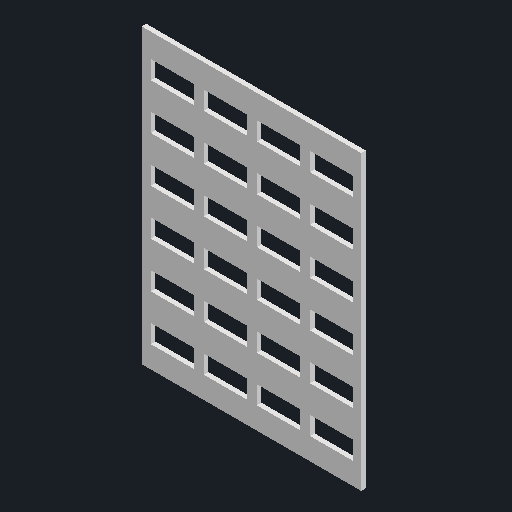
# Autodesk Inventor part: Base
Saved by Autodesk Inventor 2026.1 (Build 301233000, 233)
## iProperties
Created: 2026-06-15
Part Number: Base
Material: Generic
Document SubType Name: Modeling
Designer: aleja
Density: 1 g/cm^3
Appearance: Default
Author: aleja
Autodesk Inventor part; units mm, degrees
ref_plane "YZ Plane" through (0, 0, 0) normal (1, 0, 0) x (0, 1, 0)
ref_plane "XZ Plane" through (0, 0, 0) normal (0, 1, 0) x (-1, 0, 0)
ref_plane "XY Plane" through (0, 0, 0) normal (0, 0, 1) x (1, 0, 0)
sketch "Sketch1" plane through (0, 0, 0) normal (0, 1, 0) x (-1, 0, 0)
  line L0 (-60, 80) -> (60, 80)
  line L1 (60, 80) -> (60, -80)
  line L2 (60, -80) -> (-60, -80)
  line L3 (-60, -80) -> (-60, 80)
  line L4 (-60, 80) -> (60, -80) construction
  line L5 (60, 80) -> (-60, -80) construction
  point P0 (0, 0)
  dimension "d0" = 160
  dimension "d1" = 120
  constraints: 12 end point, 2 midpoint, 2 parallel, 1 horizontal, 1 perpendicular
  measures "d0" distance of L0.end L1.end
  measures "d1" distance of L1.end L2.end
extrude "Extrusion1" add sketch "Sketch1" along normal blind 5
sketch "Sketch2" plane through (60, 0, 80) normal (1, 0, 0) x (0, 0, -1)
  line L0 (0, 0) -> (0, 5) projected
  line L1 (0, 0) -> (0, 5) projected
  line L2 (0, 0) -> (160, 0) projected
  line L3 (160, 0) -> (160, 5) projected
  line L4 (0, 5) -> (160, 5) projected
  line L5 (0, 0) -> (0, 5) projected
  line L6 (0, 0) -> (0, 5) projected
  line L7 (0, 2.5) -> (160, 2.5)
  circle A0 centre (5, 2.5) radius 2.5
  circle A1 centre (30, 2.5) radius 2.5
  circle A2 centre (55, 2.5) radius 2.5
  circle A3 centre (80, 2.5) radius 2.5
  circle A4 centre (105, 2.5) radius 2.5
  circle A5 centre (130, 2.5) radius 2.5
  circle A6 centre (155, 2.5) radius 2.5
  point P0 (155, 5)
  point P1 (157.5, 2.5)
  point P2 (152.5, 2.5)
  point P3 (130, 5)
  point P4 (132.5, 2.5)
  point P5 (127.5, 2.5)
  point P6 (105, 5)
  point P7 (107.5, 2.5)
  point P8 (102.5, 2.5)
  point P9 (80, 5)
  point P10 (82.5, 2.5)
  point P11 (77.5, 2.5)
  point P12 (55, 5)
  point P13 (57.5, 2.5)
  point P14 (52.5, 2.5)
  point P15 (30, 5)
  point P16 (32.5, 2.5)
  point P17 (27.5, 2.5)
  point P18 (5, 5)
  point P19 (7.5, 2.5)
  point P20 (2.5, 2.5)
  point P21 (0, 5)
  dimension "d27" = 5
  dimension "d30" = 25
  constraints: 7 centre point, 2 end point, 2 midpoint, 1 horizontal, 1 point on line, 1 tangent, 12 other
  measures "d27" distance from line of L0 A0.centre
  measures "d30" distance of A0.centre A1.centre
extrude "Extrusion2" cut sketch "Sketch2" against normal through all contours L0 L4 A0 L7 | A0 L4 A1 L7 | A1 L4 A2 L7 | A2 L4 A3 L7 | A3 L4 A4 L7 | A4 L4 A5 L7 | A5 L4 A6 L7 | A6 L4 L3 L7
sketch "Sketch3" plane through (-60, 0, 80) normal (0, 0, 1) x (1, 0, 0)
  line L0 (0, 2.5) -> (0, 2.5) projected
  line L1 (120, 2.5) -> (0, 2.5) projected
  line L2 (120, 2.5) -> (120, 2.5) projected
  line L3 (120, 2.5) -> (0, 2.5) projected
  line L4 (120, 2.5) -> (0, 2.5) projected
  line L5 (0, 0) -> (0, 2.5) projected
  line L6 (0, 0) -> (120, 0) projected
  line L7 (120, 0) -> (120, 2.5) projected
  line L8 (0, 5) -> (0, 2.5) projected
  line L9 (120, 2.5) -> (120, 5) projected
  line L10 (0, 2.5) -> (120, 2.5)
  line L11 (120, 2.5) -> (120, 5)
  line L12 (120, 5) -> (0, 5)
  line L13 (0, 5) -> (0, 2.5)
  circle A0 centre (5, 2.5) radius 2.5
  circle A1 centre (15, 2.5) radius 2.5
  circle A2 centre (25, 2.5) radius 2.5
  circle A3 centre (35, 2.5) radius 2.5
  circle A4 centre (45, 2.5) radius 2.5
  circle A5 centre (55, 2.5) radius 2.5
  circle A6 centre (65, 2.5) radius 2.5
  circle A7 centre (75, 2.5) radius 2.5
  circle A8 centre (85, 2.5) radius 2.5
  circle A9 centre (95, 2.5) radius 2.5
  circle A10 centre (105, 2.5) radius 2.5
  circle A11 centre (115, 2.5) radius 2.5
  point P0 (115, 5)
  point P1 (117.5, 2.5)
  point P2 (112.5, 2.5)
  point P3 (105, 5)
  point P4 (107.5, 2.5)
  point P5 (102.5, 2.5)
  point P6 (95, 5)
  point P7 (97.5, 2.5)
  point P8 (92.5, 2.5)
  point P9 (85, 5)
  point P10 (87.5, 2.5)
  point P11 (82.5, 2.5)
  point P12 (75, 5)
  point P13 (77.5, 2.5)
  point P14 (72.5, 2.5)
  point P15 (65, 5)
  point P16 (67.5, 2.5)
  point P17 (62.5, 2.5)
  point P18 (55, 5)
  point P19 (57.5, 2.5)
  point P20 (52.5, 2.5)
  point P21 (45, 5)
  point P22 (47.5, 2.5)
  point P23 (42.5, 2.5)
  point P24 (35, 5)
  point P25 (37.5, 2.5)
  point P26 (32.5, 2.5)
  point P27 (25, 5)
  point P28 (27.5, 2.5)
  point P29 (22.5, 2.5)
  point P30 (15, 5)
  point P31 (17.5, 2.5)
  point P32 (12.5, 2.5)
  point P33 (5, 5)
  point P34 (7.5, 2.5)
  point P35 (2.5, 2.5)
  dimension "d35" = 5
  dimension "d38" = 10
  constraints: 12 centre point, 11 equal radius, 11 horizontal alignment, 8 end point, 2 parallel, 1 horizontal, 1 perpendicular, 1 point on line, 1 tangent, 1 other
  measures "d35" distance of A0.centre L0.end
  measures "d38" distance of A0.centre A1.centre
extrude "Extrusion3" cut sketch "Sketch3" against normal through all contours L1 A11 L12 L9 | L1 A10 L12 A11 | A10 L1 A9 L12 | A9 L1 A8 L12 | A8 L1 A7 L12 | A7 L1 A6 L12 | A6 L1 A5 L12 | A5 L1 A4 L12 | A4 L1 A3 L12 | A3 L1 A2 L12 | A2 L1 A1 L12 | A1 L1 A0 L12 | A0 L1 L8 L12
sketch "Sketch4" plane through (60, 2.5, 80) normal (0, 1, 0) x (1, 0, 0)
  line L0 (-115, 148) -> (-91.25, 148)
  line L1 (-91.25, 148) -> (-91.25, 138)
  line L2 (-91.25, 138) -> (-115, 138)
  line L3 (-115, 138) -> (-115, 148)
  line L4 (-120, 0) -> (-120, 160) projected
  line L5 (0, 160) -> (0, 0) projected
  line L6 (-120, 160) -> (0, 160) projected
  line L7 (-86, 148) -> (-62.25, 148)
  line L8 (-86, 138) -> (-86, 148)
  line L9 (-62.25, 138) -> (-86, 138)
  line L10 (-62.25, 148) -> (-62.25, 138)
  line L11 (-57, 148) -> (-33.25, 148)
  line L12 (-57, 138) -> (-57, 148)
  line L13 (-33.25, 138) -> (-57, 138)
  line L14 (-33.25, 148) -> (-33.25, 138)
  line L15 (-28, 148) -> (-4.25, 148)
  line L16 (-28, 138) -> (-28, 148)
  line L17 (-4.25, 138) -> (-28, 138)
  line L18 (-4.25, 148) -> (-4.25, 138)
  line L19 (-115, 123) -> (-91.25, 123)
  line L20 (-115, 113) -> (-115, 123)
  line L21 (-91.25, 113) -> (-115, 113)
  line L22 (-91.25, 123) -> (-91.25, 113)
  line L23 (-86, 123) -> (-62.25, 123)
  line L24 (-86, 113) -> (-86, 123)
  line L25 (-62.25, 113) -> (-86, 113)
  line L26 (-62.25, 123) -> (-62.25, 113)
  line L27 (-57, 123) -> (-33.25, 123)
  line L28 (-57, 113) -> (-57, 123)
  line L29 (-33.25, 113) -> (-57, 113)
  line L30 (-33.25, 123) -> (-33.25, 113)
  line L31 (-28, 123) -> (-4.25, 123)
  line L32 (-28, 113) -> (-28, 123)
  line L33 (-4.25, 113) -> (-28, 113)
  line L34 (-4.25, 123) -> (-4.25, 113)
  line L35 (-115, 98) -> (-91.25, 98)
  line L36 (-115, 88) -> (-115, 98)
  line L37 (-91.25, 88) -> (-115, 88)
  line L38 (-91.25, 98) -> (-91.25, 88)
  line L39 (-86, 98) -> (-62.25, 98)
  line L40 (-86, 88) -> (-86, 98)
  line L41 (-62.25, 88) -> (-86, 88)
  line L42 (-62.25, 98) -> (-62.25, 88)
  line L43 (-57, 98) -> (-33.25, 98)
  line L44 (-57, 88) -> (-57, 98)
  line L45 (-33.25, 88) -> (-57, 88)
  line L46 (-33.25, 98) -> (-33.25, 88)
  line L47 (-28, 98) -> (-4.25, 98)
  line L48 (-28, 88) -> (-28, 98)
  line L49 (-4.25, 88) -> (-28, 88)
  line L50 (-4.25, 98) -> (-4.25, 88)
  line L51 (-115, 73) -> (-91.25, 73)
  line L52 (-115, 63) -> (-115, 73)
  line L53 (-91.25, 63) -> (-115, 63)
  line L54 (-91.25, 73) -> (-91.25, 63)
  line L55 (-86, 73) -> (-62.25, 73)
  line L56 (-86, 63) -> (-86, 73)
  line L57 (-62.25, 63) -> (-86, 63)
  line L58 (-62.25, 73) -> (-62.25, 63)
  line L59 (-57, 73) -> (-33.25, 73)
  line L60 (-57, 63) -> (-57, 73)
  line L61 (-33.25, 63) -> (-57, 63)
  line L62 (-33.25, 73) -> (-33.25, 63)
  line L63 (-28, 73) -> (-4.25, 73)
  line L64 (-28, 63) -> (-28, 73)
  line L65 (-4.25, 63) -> (-28, 63)
  line L66 (-4.25, 73) -> (-4.25, 63)
  line L67 (-115, 48) -> (-91.25, 48)
  line L68 (-115, 38) -> (-115, 48)
  line L69 (-91.25, 38) -> (-115, 38)
  line L70 (-91.25, 48) -> (-91.25, 38)
  line L71 (-86, 48) -> (-62.25, 48)
  line L72 (-86, 38) -> (-86, 48)
  line L73 (-62.25, 38) -> (-86, 38)
  line L74 (-62.25, 48) -> (-62.25, 38)
  line L75 (-57, 48) -> (-33.25, 48)
  line L76 (-57, 38) -> (-57, 48)
  line L77 (-33.25, 38) -> (-57, 38)
  line L78 (-33.25, 48) -> (-33.25, 38)
  line L79 (-28, 48) -> (-4.25, 48)
  line L80 (-28, 38) -> (-28, 48)
  line L81 (-4.25, 38) -> (-28, 38)
  line L82 (-4.25, 48) -> (-4.25, 38)
  line L83 (-115, 23) -> (-91.25, 23)
  line L84 (-115, 13) -> (-115, 23)
  line L85 (-91.25, 13) -> (-115, 13)
  line L86 (-91.25, 23) -> (-91.25, 13)
  line L87 (-86, 23) -> (-62.25, 23)
  line L88 (-86, 13) -> (-86, 23)
  line L89 (-62.25, 13) -> (-86, 13)
  line L90 (-62.25, 23) -> (-62.25, 13)
  line L91 (-57, 23) -> (-33.25, 23)
  line L92 (-57, 13) -> (-57, 23)
  line L93 (-33.25, 13) -> (-57, 13)
  line L94 (-33.25, 23) -> (-33.25, 13)
  line L95 (-28, 23) -> (-4.25, 23)
  line L96 (-28, 13) -> (-28, 23)
  line L97 (-4.25, 13) -> (-28, 13)
  line L98 (-4.25, 23) -> (-4.25, 13)
  point P0 (-60, 80)
  dimension "d43" = 5
  dimension "d44" = 23.75
  dimension "d45" = 120
  dimension "d46" = 10
  dimension "d47" = 12
  dimension "d50" = 29
  dimension "d53" = 25
  constraints: 192 end point, 2 collinear, 2 horizontal, 2 parallel, 1 perpendicular, 1 vertical, 182 other
  measures "d43" distance between parallel lines of L4 L3
  measures "d44" distance of L0.start L0.end
  measures "d45" distance from line of L5 L4.end
  measures "d46" distance of L2.end L0.start
  measures "d47" distance between parallel lines of L6 L0
  measures "d50" distance of L0.start L7.start
  measures "d53" distance of L0.start L19.start
extrude "Extrusion4" cut sketch "Sketch4" against normal blind 10
body "Solid1"
